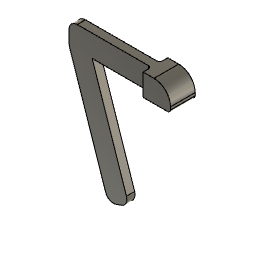
arm (Autodesk Fusion 360 design; units mm, degrees)
Autodesk Fusion 360 part; units mm, degrees
sketch "Sketch1" plane through (0, 0, 0) normal (0, 1, 0) x (1, 0, 0)
  line L0 (0, 0) -> (40, 0)
  line L1 (40, 0) -> (40, -8)
  line L2 (40, -8) -> (0, -8)
  line L3 (0, -8) -> (0, 0)
  line L4 (0, 0) -> (14.3059, 42.6654)
  line L5 (14.3059, 42.6654) -> (21.8909, 40.1222)
  line L6 (21.8909, 40.1222) -> (8.4377, 0)
  dimension "d1" = 40
  dimension "d2" = 8
  dimension "d4" = 8
  dimension "d5" = 71.463
  dimension "d9" = 45
  constraint horizontal L0
  constraint vertical L1
  constraint horizontal L2
  constraint vertical L3
  constraint coincident L0.start L3.end
  constraint perpendicular L4 L5
  constraint coincident L0 L6.end
  constraint perpendicular L5 L6
  measures "d1" distance of L0.start L0.end
  measures "d2" distance of L0.start L2.end
  measures "d4" distance of L4 L6
  measures "d5" angle of L0 L6
  measures "d9" distance of L0.start L4.end
extrude "Extrude3" add sketch "Sketch1" along normal blind 3
fillet "Fillet8" radius 3 4 edges at (0, 1.5, 8) (0, 1.5, 0) (14.3059, 1.5, -42.6654) (21.8909, 1.5, -40.1222)
sketch "Sketch4" plane through (0, 0, 0) normal (0, -1, 0) x (1, 0, 0)
  arc A0 (19.0465, -41.0759) -> (20.9372, -37.2778) centre (18.0928, -38.2315) ccw
  line L0 (20.9372, -37.2778) -> (8.4377, 0)
  line L1 (8.4377, 0) -> (40, 0)
  line L2 (40, 0) -> (40, 8)
  line L3 (40, 8) -> (3, 8)
  arc A1 (3, 8) -> (0, 5) centre (3, 5) ccw
  line L4 (0, 5) -> (0, 0.4896)
  arc A2 (0, 0.4896) -> (0.1556, -0.4642) centre (3, 0.4896) ccw
  line L5 (0.1556, -0.4642) -> (13.3522, -39.8211)
  arc A3 (13.3522, -39.8211) -> (17.1503, -41.7117) centre (16.1966, -38.8674) ccw
  line L6 (17.1503, -41.7117) -> (19.0465, -41.0759)
  line L7 (40, 8) -> (30, 8)
  line L8 (30, 8) -> (30, 0)
  line L9 (30, 0) -> (40, 0)
  line L10 (40, 0) -> (40, 8)
  dimension "d26" = 10
  constraint horizontal L7
  constraint vertical L8
  constraint horizontal L9
  constraint vertical L10
  constraint coincident L1 L8.end
  constraint coincident L2.end L3.start
  measures "d26" distance of L8 L10
extrude "Extrude4" add sketch "Sketch4" along normal blind 3 and the other way blind 6 contours L1 L2 L3 L7 L8 L9 L10
fillet "Fillet9" radius 6 1 edges at (40, 1.5, 8)
fillet "Fillet10" radius 1 1 edges at (40, 1.5, 0)
fillet "Fillet11" radius 1 2 edges at (30, 0, 4) (30, 3, 4)
extrude "Extrude1" [suppressed]
moveface "MoveFace1" [suppressed]
fillet "Fillet1" [suppressed]
fillet "Fillet2" [suppressed]
sketch "Sketch2" plane through (0, 0, 0) normal (0, 1, 0) x (1, 0, 0)
  line L0 (40, -8) -> (31, -8)
  line L1 (31, -8) -> (31, 0)
  line L2 (31, 0) -> (40, 0)
  line L3 (40, 0) -> (40, -8)
  line L4 (40, 0) -> (40, -8)
  dimension "d12" = 9
  dimension "d13" = 8
  constraint horizontal L0
  constraint vertical L1
  constraint horizontal L2
  constraint vertical L3
  measures "d12" distance of L1 L4
  measures "d13" distance of L0 L2
extrude "Extrude2" [suppressed]
fillet "Fillet3" [suppressed]
fillet "Fillet4" [suppressed]
fillet "Fillet5" [suppressed]
sketch "Sketch3" plane through (0, 0, 0) normal (0, 1, 0) x (1, 0, 0)
delete_face "DeleteFace1" [suppressed]
fillet "Fillet6" [suppressed]
delete_face "DeleteFace2" [suppressed]
fillet "Fillet7" [suppressed]
